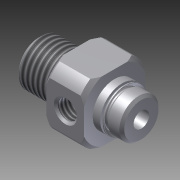
# Autodesk Inventor part: 007R000_rod_guide
Saved by Autodesk Inventor 2012 (Build 160160000, 160)
## iProperties
Created: 2013-01-17
Part Number: 007R000_rod_guide
Material: Default
Catalog Web Link: www.cadenas.de
Description: Rod Guide-Original Line - Standard Air Cylinders
Vendor: BIMBA
Document SubType Name: Modeling
Designer: William
Manufacturer: BIMBA
Density: 1 g/cm^3
Category: PARTsolutions
Company: BIMBA
Title: 007R000_rod_guide
Author: Cadenas PARTsolutions
Comments: Original Line - Standard Air Cylinders
PSOL_IDENT_0: {\\10.0.0.242\data_v9\23d-libs\bimba\bimba\bimba_imperial\bimba_full_line\original_line_cylinders\st
PSOL_IDENT_1: andard_air_cylinders\rod_guide.prj},221 {VTYP=3D},{NB=007R000_rod_guide},{LINA=007R000_rod_guide},{N
PSOL_IDENT_2: N=Rod Guide},{DATE=11.09.2012 04:45:35},{GEOMDATE=11.09.2012 04:45:00},{VERSION=},{LINEID=10},{LINES
PSOL_IDENT_3: UBID=-1},{WBVAR=MNT,ACTING,NR,K,Q,T1,T2,T3,T4,MB,TRIM,CUSH}  {NB=007R000_rod_guide},{LINA=007R000_ro
PSOL_IDENT_4: d_guide},{KT=DUMMY},{PN=007R000},{BORE=0.31250000},{BOREPN=007},{MNT=},{MNTALG='' , 'Front Nose' , '
PSOL_IDENT_5: BF' , 'Front Block'},{ACTING=R},{ACTINGALG= '' , 'Single Acting' , 'R' , 'Reverse/Double Acting' },{
PSOL_IDENT_6: NR=},{NRALG= '' , 'N/A' },{K=},{Q=},{QALG= '' , 'Without Side Ported Rear Head' , 'Q' , 'With Side P
PSOL_IDENT_7: orted Rear Head' },{T1=},{T2=},{T3=},{T4=},{MB=0},{A1=0.8450},{A1N=0.6250},{A1P=0.8450},{A1B=0.9060}
PSOL_IDENT_8: ,{A2=0.3120},{A2N=0.2500},{A2P=0.3120},{A3=0.3125},{A3N=0.1200},{A3P=0.3125},{A4=0.1585},{A4N=0.2550
PSOL_IDENT_9: },{A4P=0.1585},{A5=0.0220},{A6=0.0000},{A6N=0.1025},{A6P=0.0000},{A7=0.3040},{A7N=0.2050},{A7P=0.304
PSOL_IDENT_10: 0},{A8=0.0150},{A8N=0.0150},{A8NR=0.0150},{D1=0.6050},{D1N=0.3590},{D1P=0.6050},{D1B=0.0000},{D2=0.3
PSOL_IDENT_11: 215},{D3=0.0000},{D3N=0.2350},{D3P=0.0000},{D4=0.1530},{D4N=0.1420},{D4P=0.1530},{D4NR=0.1530},{D5=0
PSOL_IDENT_12: .1280},{D5N=0.1280},{D5NR=0.1280},{C1=0.020},{C2=0.0200},{C2N=0.0200},{C2P=0.0200},{C3=0.0300},{C3N=
PSOL_IDENT_13: 0.0000},{C3P=0.0300},{C4=0.0300},{C4N=0.0200},{C4P=0.0300},{NDM=0.3750},{NDMN=0.2500},{NDMP=0.3750},
PSOL_IDENT_14: {TAB=UNF},{D6=0.0000},{D6N=0.0000},{D6P=0.0000},{A9=0.0000},{A9N=0.0000},{A9P=0.0000},{D7=0.0000},{D
PSOL_IDENT_15: 7N=0.0000},{D7P=0.0000},{A10=0.0000},{A10N=0.0000},{A10P=0.0000},{R1=0.0000},{R1N=0.0000},{R1P=0.000
PSOL_IDENT_16: 0},{D8=0.0000},{D9=0.0000},{D10=0.0000},{A11=0.0000},{A12=0.0000},{A13=0.0000},{A14=0.3750},{A14N=0.
PSOL_IDENT_17: 3750},{A14B=0.5000},{D11=0.0000},{D11N=0.0000},{NDM2=0.1900},{NDM2N=0.1900},{NDM2DP=0.0000},{THREAD=
PSOL_IDENT_18: 1},{HEX=0.0000},{HEXN=0.0000},{S1=0.5000},{B1=0.0620},{B2=0.5940},{B22=0.0000},{DB=0.1130},{B3=0.015
PSOL_IDENT_19: 0},{B4=0.3430},{X1=0.0000},{X2=0.0000},{NDM3=0.0000},{NDM4=0.0000},{NDM4DP=0.0000},{DD=0.0000},{CB=0
PSOL_IDENT_20: .0000},{CBDP=0.0000},{PORT=1},{XT=0.0000},{XTX=0.0000},{XT1=0.0000},{XT2=0.0000},{NDMH=0.0000},{OD=0
PSOL_IDENT_21: .3590},{ID=0.3215},{G=0.0000},{PNUT=0.3120},{TRIM=0},{C11=0.0000},{C22=0.0000},{C33=0.0000},{C44=0.0
PSOL_IDENT_22: 000},{C55=0.0000},{CD1=0.0000},{CD2=0.0000},{CD3=0.0000},{CNDM3=0.0000},{CTAB3=0.0000},{CUSH=0},{XX=
PSOL_IDENT_23: 0.34300},{LCD=0.0000}
CNS_NT: Original Line - Standard Air Cylinders
CNS_NB: 007R000_rod_guide
CNS_NBSYN: $PN._rod_guide
CNS_LINA: 007R000_rod_guide
CNS_PN: 007R000
CNS_BORE: 5/16
CNS_BOREPN: 007
CNS_MNT: Front Nose
CNS_MNTALG: '' , 'Front Nose' , 'BF' , 'Front Block'
CNS_ACTING: Reverse/Double Acting
CNS_ACTINGALG: '' , 'Single Acting' , 'R' , 'Reverse/Double Acting'
CNS_NR: N/A
CNS_NRALG: '' , 'N/A'
CNS_K: Standard
CNS_Q: Without Side Ported Rear Head
CNS_QALG: '' , 'Without Side Ported Rear Head' , 'Q' , 'With Side Ported Rear Head'
CNS_T1: without T1
CNS_T2: without T2
CNS_T3: without T3
CNS_T4: without T4
CNS_MB: 0
CNS_A1: 0.8450
CNS_A1N: 0.6250
CNS_A1P: 0.8450
CNS_A1B: 0.9060
CNS_A2: 0.3120
CNS_A2N: 0.2500
CNS_A2P: 0.3120
CNS_A3: 0.3125
CNS_A3N: 0.1200
CNS_A3P: 0.3125
CNS_A4: 0.1585
CNS_A4N: 0.2550
CNS_A4P: 0.1585
CNS_A5: 0.0220
CNS_A6: 0.0000
CNS_A6N: 0.1025
CNS_A6P: 0.0000
CNS_A7: 0.3040
CNS_A7N: 0.2050
CNS_A7P: 0.3040
CNS_A8: 0.0150
CNS_A8N: 0.0150
CNS_A8NR: 0.0150
CNS_D1: 0.6050
CNS_D1N: 0.3590
CNS_D1P: 0.6050
CNS_D1B: 0.0000
CNS_D2: 0.3215
CNS_D3: 0.0000
CNS_D3N: 0.2350
CNS_D3P: 0.0000
CNS_D4: 0.1530
CNS_D4N: 0.1420
CNS_D4P: 0.1530
CNS_D4NR: 0.1530
CNS_D5: 0.1280
CNS_D5N: 0.1280
CNS_D5NR: 0.1280
CNS_C1: 0.020
CNS_C2: 0.0200
CNS_C2N: 0.0200
CNS_C2P: 0.0200
CNS_C3: 0.0300
CNS_C3N: 0.0000
CNS_C3P: 0.0300
CNS_C4: 0.0300
CNS_C4N: 0.0200
CNS_C4P: 0.0300
CNS_NDM: 0.3750
CNS_NDMN: 0.2500
CNS_NDMP: 0.3750
CNS_TAB: UNF
CNS_D6: 0.0000
CNS_D6N: 0.0000
CNS_D6P: 0.0000
CNS_A9: 0.0000
CNS_A9N: 0.0000
CNS_A9P: 0.0000
CNS_D7: 0.0000
CNS_D7N: 0.0000
CNS_D7P: 0.0000
CNS_A10: 0.0000
CNS_A10N: 0.0000
CNS_A10P: 0.0000
CNS_R1: 0.0000
CNS_R1N: 0.0000
CNS_R1P: 0.0000
CNS_D8: 0.0000
CNS_D9: 0.0000
CNS_D10: 0.0000
CNS_A11: 0.0000
CNS_A12: 0.0000
CNS_A13: 0.0000
CNS_A14: 0.3750
CNS_A14N: 0.3750
CNS_A14B: 0.5000
CNS_D11: 0.0000
CNS_D11N: 0.0000
CNS_NDM2: 0.1900
CNS_NDM2N: 0.1900
CNS_NDM2DP: 0.0000
CNS_THREAD: 1
CNS_HEX: 0.0000
CNS_HEXN: 0.0000
CNS_S1: 0.5000
CNS_B1: 0.0620
CNS_B2: 0.5940
CNS_B22: 0.0000
CNS_DB: 0.1130
CNS_B3: 0.0150
CNS_B4: 0.3430
CNS_X1: 0.0000
CNS_X2: 0.0000
CNS_NDM3: 0.0000
CNS_NDM4: 0.0000
CNS_NDM4DP: 0.0000
CNS_DD: 0.0000
CNS_CB: 0.0000
CNS_CBDP: 0.0000
CNS_PORT: 1
CNS_XT: 0.0000
CNS_XTX: 0.0000
CNS_XT1: 0.0000
CNS_XT2: 0.0000
CNS_NDMH: 0.0000
CNS_OD: 0.3590
CNS_ID: 0.3215
CNS_G: 0.0000
CNS_PNUT: 0.3120
CNS_TRIM: 0
CNS_C11: 0.0000
CNS_C22: 0.0000
CNS_C33: 0.0000
CNS_C44: 0.0000
CNS_C55: 0.0000
CNS_CD1: 0.0000
CNS_CD2: 0.0000
CNS_CD3: 0.0000
CNS_CNDM3: 0.0000
CNS_CTAB3: 0.0000
CNS_CUSH: 0
CNS_XX: 0.34300
CNS_LCD: 0.0000
SUPPLIER: BIMBA
ARTICLENO: 007R000_rod_guide
BOMINFO: 007R000_rod_guide
CREATOR: CADENAS GmbH
Autodesk Inventor part; units mm, degrees
sketch "Sketch_1" plane through (0, 0, 0) normal (0, 0, 1) x (1, 0, 0)
  line L0 (7.9248, 0) -> (0, 0)
  line L1 (0, 0) -> (0, 4.1326)
  line L2 (0, 4.1326) -> (0.6299, 4.7625)
  line L3 (0.6299, 4.7625) -> (7.9248, 4.7625)
  line L4 (7.9248, 4.7625) -> (7.9248, 0)
  line L5 (7.9248, 0) -> (0, 0)
  constraints: 12 end point
revolve "Revolution1" add sketch "Sketch_1" angle 360 about axis through (7.9248, 0, 0) along (1, 0, 0)
thread "Thread1" size "3/8-24 UNF" class "2A" standard "ANSI Unified Screw Threads" full length
sketch "Sketch_3" plane through (0, 0, 0) normal (0, 0, 1) x (1, 0, 0)
  line L0 (21.463, 0) -> (7.9248, 0)
  line L1 (7.9248, 0) -> (7.9248, 6.9215)
  line L2 (7.9248, 6.9215) -> (8.6868, 7.6835)
  line L3 (8.6868, 7.6835) -> (15.1003, 7.6835)
  line L4 (15.1003, 7.6835) -> (15.8623, 6.9215)
  line L5 (15.8623, 6.9215) -> (15.8623, 3.5242)
  line L6 (15.8623, 3.5242) -> (17.9959, 3.5242)
  line L7 (17.9959, 3.5242) -> (18.5547, 4.0831)
  line L8 (18.5547, 4.0831) -> (20.955, 4.0831)
  line L9 (20.955, 4.0831) -> (21.463, 3.5751)
  line L10 (21.463, 3.5751) -> (21.463, 0)
  line L11 (21.463, 0) -> (7.9248, 0)
  constraints: 24 end point
revolve "Revolution2" add sketch "Sketch_3" angle 360 about axis through (21.463, 0, 0) along (1, 0, 0)
sketch "Sketch_17" plane through (0, 0, 0) normal (0, 0, 1) x (1, 0, 0)
  line L0 (17.4371, 0) -> (15.8623, 0)
  line L1 (15.8623, 0) -> (15.8623, 4.5593)
  line L2 (15.8623, 4.5593) -> (17.4371, 4.5593)
  line L3 (17.4371, 4.5593) -> (17.4371, 0)
  line L4 (17.4371, 0) -> (15.8623, 0)
  constraints: 10 end point
revolve "Revolution3" add sketch "Sketch_17" angle 360 about axis through (17.4371, 0, 0) along (1, 0, 0)
sketch "Sketch4" plane through (0, 0, 0) normal (-1, 0, 0) x (0, 0, 1)
  point P0 (0, 0)
hole "Drilling 1" at (0, 0, 0) direction (1, 0, 0) diameter 3.2512 depth 21.463 countersink diameter 4.0132 countersink angle 90
sketch "Sketch_16" plane through (0, 0, 0) normal (1, 0, 0) x (0, 1, 0)
  line L0 (12.7, 12.7) -> (-12.7, 12.7)
  line L1 (-12.7, 12.7) -> (-12.7, -12.7)
  line L2 (-12.7, -12.7) -> (12.7, -12.7)
  line L3 (12.7, -12.7) -> (12.7, 12.7)
  line L4 (6.35, 6.35) -> (-6.35, 6.35)
  line L5 (-6.35, 6.35) -> (-6.35, -6.35)
  line L6 (-6.35, -6.35) -> (6.35, -6.35)
  line L7 (6.35, -6.35) -> (6.35, 6.35)
  constraints: 16 end point
extrude "Extrusion1" cut sketch "Sketch_16" along normal blind 21.463
sketch "Sketch6" plane through (8.6868, -4.3259, 6.35) normal (0, 0, 1) x (1, 0, 0)
  point P0 (3.2512, 4.3259)
hole "Drilling 2" at (11.938, 0, 6.35) direction (0, 0, -1) diameter 3.9624 depth 6.35 countersink diameter 4.826 countersink angle 90 thread size "10-32 UNF" class "2B" standard "ANSI Unified Screw Threads"
sketch "Sketch_47" plane through (0, 0, 0) normal (0, 0, 1) x (1, 0, 0)
  line L0 (17.9959, 0) -> (17.4371, 0)
  line L1 (17.4371, 3.2702) -> (17.9959, 3.2702)
  line L2 (17.9959, 3.2702) -> (17.9959, 3.5242)
  line L3 (17.9959, 3.5242) -> (17.7165, 3.5242)
  line L4 (17.7165, 3.5242) -> (17.5509, 3.6899)
  arc A0 (17.5509, 3.8695) -> (17.5509, 3.6899) centre (17.6407, 3.7797) ccw
  line L5 (17.5509, 3.8695) -> (18.1565, 4.4751)
  line L6 (18.1565, 4.4751) -> (18.1565, 4.5593)
  line L7 (18.1565, 4.5593) -> (17.9533, 4.5593)
  line L8 (17.9533, 4.5593) -> (17.4371, 4.0431)
  line L9 (17.4371, 4.0431) -> (17.4371, 3.2702)
  constraints: 20 end point, 2 point on circle, 1 centre point
revolve "Revolution4" add sketch "Sketch_47" angle 360 about axis through (17.9959, 0, 0) along (1, 0, 0)
ref_plane "sq1_XY" through (0, 0, 6.35) normal (1, 0, 0) x (0, 0, -1)
ref_plane "sq1_YZ" through (0, 0, 6.35) normal (0, 0, -1) x (0, 1, 0)
ref_plane "sq1_ZX" through (0, 0, 6.35) normal (0, 1, 0) x (1, 0, 0)
ref_plane "sq2_XY" through (0, 0, -6.35) normal (1, 0, 0) x (0, 0, -1)
ref_plane "sq2_YZ" through (0, 0, -6.35) normal (0, 0, -1) x (0, 1, 0)
ref_plane "sq2_ZX" through (0, 0, -6.35) normal (0, 1, 0) x (1, 0, 0)
ref_plane "rod_guide_XY" through (0, 0, 0) normal (1, 0, 0) x (0, 0, -1)
ref_plane "rod_guide_YZ" through (0, 0, 0) normal (0, 0, -1) x (0, 1, 0)
ref_plane "rod_guide_ZX" through (0, 0, 0) normal (0, 1, 0) x (1, 0, 0)
ref_plane "to_tube_XY" through (17.9959, 0, 0) normal (1, 0, 0) x (0, 0, -1)
ref_plane "to_tube_YZ" through (17.9959, 0, 0) normal (0, 0, -1) x (0, 1, 0)
ref_plane "to_tube_ZX" through (17.9959, 0, 0) normal (0, 1, 0) x (1, 0, 0)
ref_plane "to_foot_bracket_XY" through (7.9248, 0, 0) normal (1, 0, 0) x (0, 0, -1)
ref_plane "to_foot_bracket_YZ" through (7.9248, 0, 0) normal (0, 0, -1) x (0, 1, 0)
ref_plane "to_foot_bracket_ZX" through (7.9248, 0, 0) normal (0, 1, 0) x (1, 0, 0)
ref_plane "to_nut_XY" through (7.9248, 0, 0) normal (1, 0, 0) x (0, 0, -1)
ref_plane "to_nut_YZ" through (7.9248, 0, 0) normal (0, 0, -1) x (0, 1, 0)
ref_plane "to_nut_ZX" through (7.9248, 0, 0) normal (0, 1, 0) x (1, 0, 0)
ref_plane "to_trunnion_brackets_XY" through (0, 0, 0) normal (0, 1, 0) x (1, 0, 0)
ref_plane "to_trunnion_brackets_YZ" through (0, 0, 0) normal (1, 0, 0) x (0, 0, -1)
ref_plane "to_trunnion_brackets_ZX" through (0, 0, 0) normal (0, 0, -1) x (0, 1, 0)
ref_plane "to_trunnion_brackets1_XY" through (0, 6.35, 0) normal (0, 1, 0) x (1, 0, 0)
ref_plane "to_trunnion_brackets1_YZ" through (0, 6.35, 0) normal (1, 0, 0) x (0, 0, -1)
ref_plane "to_trunnion_brackets1_ZX" through (0, 6.35, 0) normal (0, 0, -1) x (0, 1, 0)
ref_plane "to_trunnion_brackets2_XY" through (0, -6.35, 0) normal (0, 1, 0) x (1, 0, 0)
ref_plane "to_trunnion_brackets2_YZ" through (0, -6.35, 0) normal (1, 0, 0) x (0, 0, -1)
ref_plane "to_trunnion_brackets2_ZX" through (0, -6.35, 0) normal (0, 0, -1) x (0, 1, 0)
ref_plane "t111_XY" through (7.9248, 0, 0) normal (1, 0, 0) x (0, 0, -1)
ref_plane "t111_YZ" through (7.9248, 0, 0) normal (0, 0, -1) x (0, 1, 0)
ref_plane "t111_ZX" through (7.9248, 0, 0) normal (0, 1, 0) x (1, 0, 0)
ref_plane "t1_XY" through (7.9248, 0, 0) normal (1, 0, 0) x (0, 0, -1)
ref_plane "t1_YZ" through (7.9248, 0, 0) normal (0, 0, -1) x (0, 1, 0)
ref_plane "t1_ZX" through (7.9248, 0, 0) normal (0, 1, 0) x (1, 0, 0)
ref_plane "port_XY" through (11.938, 0, 0) normal (0, 0, 1) x (1, 0, 0)
ref_plane "port_YZ" through (11.938, 0, 0) normal (1, 0, 0) x (0, 1, 0)
ref_plane "port_ZX" through (11.938, 0, 0) normal (0, 1, 0) x (0, 0, 1)
ref_plane "to_screw_XY" through (11.938, 0, 0) normal (0, 1, 0) x (1, 0, 0)
ref_plane "to_screw_YZ" through (11.938, 0, 0) normal (1, 0, 0) x (0, 0, -1)
ref_plane "to_screw_ZX" through (11.938, 0, 0) normal (0, 0, -1) x (0, 1, 0)
body "Solid1"
